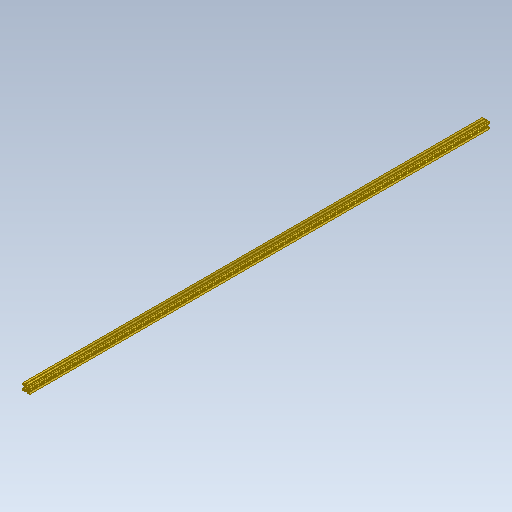
# Autodesk Inventor part: Perfil 30×30 2 rasgos opostos_AST03003002O
Saved by Autodesk Inventor 2025.2 (Build 292293000, 293)
## iProperties
Created: 2025-04-06
Part Number: Perfil 30×30 2 rasgos opostos_AST03003002O
Material: Ouro
Document SubType Name: Modeling
Designer: Gustavo Sousa
Density: 19.3 g/cm^3
Appearance: Metal quente 2400F
Author: Gustavo Sousa
Autodesk Inventor part; units mm, degrees
ref_plane "YZ Plane" through (0, 0, 0) normal (1, 0, 0) x (0, 1, 0)
ref_plane "XZ Plane" through (0, 0, 0) normal (0, 1, 0) x (-1, 0, 0)
ref_plane "XY Plane" through (0, 0, 0) normal (0, 0, 1) x (1, 0, 0)
sketch "Esboço1" plane through (0, 0, 0) normal (0, 0, 1) x (1, 0, 0)
  circle A0 centre (0, 0) radius 5 construction
  line L0 (-15, 15) -> (15, 15) construction
  arc A1 (0, 5) -> (-5, 0) centre (0, 0) ccw
  line L1 (-3.5355, 3.5355) -> (0, 0) construction
  line L2 (-3.5355, 3.5355) -> (-15, 15) construction
  line L3 (-7, 7) -> (7, 7) construction
  line L4 (-15, 15) -> (-15, -15) construction
  line L5 (-7, 7) -> (-7, -7) construction
  line L6 (-15, 4.1) -> (-15, -4.1)
  line L7 (-15, 4.1) -> (-12.8, 4.1) construction
  line L8 (-12.8, 4.1) -> (-12.8, 8.15) construction
  line L9 (-9.7056, 8.15) -> (-7, 5.4444) construction
  line L10 (-12.8, 8.15) -> (-9.7056, 8.15) construction
  line L11 (-7, 5.4444) -> (-7, 0) construction
  line L12 (-15, 4.1) -> (-14.5, 4.1) construction
  line L13 (-14.5, 4.1) -> (-14.5, 4.6)
  line L14 (-14.5, 4.6) -> (-15, 4.6)
  line L15 (-15, 4.6) -> (-15, 4.1) construction
  line L16 (-14.5, 4.1) -> (-12.8, 4.1)
  arc A2 (-14.5, 15) -> (-15, 14.5) centre (-14.5, 14.5) ccw
  line L17 (-15, 14.5) -> (-15, 4.6)
  circle A3 centre (-11.5, 11.5) radius 2.25
  line L18 (-8.15, 13.9) -> (-8.15, 9.7056) construction
  line L19 (-8.15, 9.7056) -> (-5.4444, 7) construction
  line L20 (-5.4444, 7) -> (0, 7) construction
  line L21 (-11.5, 11.5) -> (-11.5, 13.75) construction
  line L22 (-8.15, 13.9) -> (-6.7972, 13.9) construction
  line L23 (-6.7972, 13.9) -> (-6.7972, 12.8)
  line L24 (-6.7972, 12.8) -> (-4.3134, 12.8)
  line L25 (-4.3134, 12.8) -> (-4.3134, 13.9)
  line L26 (-4.3134, 13.9) -> (0, 13.9)
  circle A4 centre (-3.5355, 3.5355) radius 1.1 construction
  arc A5 (-2.6769, 4.2231) -> (-4.2231, 2.6769) centre (-3.5355, 3.5355) ccw
  line L27 (-7, 0) -> (-5, 0)
  line L28 (0, 13.9) -> (0, 15)
  arc A6 (-12.3, 8.15) -> (-12.8, 7.65) centre (-12.3, 7.65) ccw
  arc A7 (-9.5592, 8.0036) -> (-9.9127, 8.15) centre (-9.9127, 7.65) ccw
  arc A8 (-7, 5.2373) -> (-7.1464, 5.5908) centre (-7.5, 5.2373) ccw
  arc A9 (-5.5908, 7.1464) -> (-5.2373, 7) centre (-5.2373, 7.5) ccw
  arc A10 (-8.15, 9.9127) -> (-8.0036, 9.5592) centre (-7.65, 9.9127) ccw
  arc A11 (-7.65, 13.9) -> (-8.15, 13.4) centre (-7.65, 13.4) ccw
  line L29 (-12.8, 7.65) -> (-12.8, 4.1)
  line L30 (-12.3, 8.15) -> (-9.9127, 8.15)
  line L31 (-9.5592, 8.0036) -> (-7.1464, 5.5908)
  line L32 (-7, 5.2373) -> (-7, 0)
  line L33 (-6.7972, 13.9) -> (-7.65, 13.9)
  line L34 (-8.15, 13.4) -> (-8.15, 9.9127)
  line L35 (-8.0036, 9.5592) -> (-5.5908, 7.1464)
  line L36 (-5.2373, 7) -> (0, 7)
  line L37 (0, 7) -> (0, 5)
  line L38 (-14.5, 15) -> (0, 15)
  line L39 (-14.8536, 14.8536) -> (-13.091, 13.091)
  line L40 (-9.909, 9.909) -> (-4.3134, 4.3134)
  point P0 (-15, 0)
  point P1 (-15, 0)
  point P2 (-6.7972, 8.3528)
  point P3 (-12.3, 8.15)
  dimension "d0" = 10
  dimension "d1" = 15
  dimension "d2" = 30
  dimension "d3" = 8
  dimension "d5" = 8.2
  dimension "espessura" = 2.2
  dimension "d7" = 1.1
  dimension "quadrado" = 0.5
  dimension "arco" = 0.5
  dimension "d10" = 4.5
  dimension "d13" = 1.1
  dimension "d14" = 11.5
  dimension "d16" = 1.1
  dimension "d21" = 2.2
  dimension "d25" = 2.2
  dimension "d26" = 1.1
  constraints: 82 end point, 30 point on circle, 20 point on line, 15 tangent, 12 centre point, 10 collinear, 9 vertical, 7 equal radius, 6 horizontal, 6 midpoint, 5 perpendicular, 5 vertical alignment, 4 coincident, 4 equal length, 4 horizontal alignment, 4 parallel
  measures "d0" diameter of A0
  measures "d1" distance from line of point (0, 0) L0
  measures "d2" distance of L0.start L0.end
  measures "d3" distance between parallel lines of L0 L3
  measures "d5" distance of L6.start L6.end
  measures "espessura" distance between parallel lines of L4 L8
  measures "d7" distance between parallel lines of L2 L9
  measures "quadrado" distance of L13.end L14.end
  measures "arco" radius of A2
  measures "d10" diameter of A3
  measures "d13" distance edge to line of A3 L10
  measures "d14" horizontal distance of point (0, 0) L21.start
  measures "d16" distance between parallel lines of L2 L19
  measures "d21" diameter of A4
  measures "d25" distance between parallel lines of L0 L24
  measures "d26" distance between parallel lines of L0 L22
extrude "Extrusão5" add sketch "Esboço1" along normal mid plane 2000 contours A1 L27 L32 A8 L31 A7 L30 A6 L29 L16 L13 L14 L17 A2 L39 A3 L40 A5
mirror "Espelhar11" about plane through (-7, 0, 0) normal (0, -1, 0) of "Extrusão5"
mirror "Espelhar12" about plane through (0, 0, 0) normal (1, 0, 0) of "Extrusão5", "Espelhar11"
mirror "Espelhar13" about plane through (-13.091, -13.091, 0) normal (0.7071068, -0.7071068, 0) of "Extrusão5", "Espelhar11"
extrude "Extrusão6" add sketch "Esboço1" along normal mid plane 2000 contours A1 A5 L40 A3 L39 A2 L38 L28 L26 L25 L24 L23 L33 A11 L34 A10 L35 A9 L36 L37
mirror "Espelhar14" about plane through (0, 0, 0) normal (1, 0, 0) of "Extrusão6"
equation "\"d13\" = 0.5 * espessura"
equation "\"d16\" = 0.5 * espessura"
equation "\"d25\" = espessura"
equation "\"d26\" = 0.5 * espessura"
